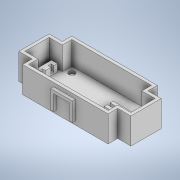
# Autodesk Inventor part: Final Design
Saved by Autodesk Inventor 2021 (Build 250183000, 183)
## iProperties
Created: 2020-11-11
Part Number: Final Design
Material: Generic
Document SubType Name: Modeling
Designer: coupe
Density: 1 g/cm^3
Appearance: Default
Mass: 94.4027 g
Surface Area: 493.885 cm^2
Volume: 94.4027 cm^3
Author: coupe
Autodesk Inventor part; units mm, degrees
ref_plane "YZ Plane" through (0, 0, 0) normal (1, 0, 0) x (0, 1, 0)
ref_plane "XZ Plane" through (0, 0, 0) normal (0, 1, 0) x (-1, 0, 0)
sketch "Sketch1" plane through (0, 0, 0) normal (0, 0, 1) x (1, 0, 0)
  line L0 (0, 0) -> (150.4, 0)
  line L1 (150.4, 0) -> (150.4, 35)
  line L2 (150.4, 35) -> (0, 35)
  line L3 (0, 35) -> (0, 0)
  line L4 (0, 35) -> (17.78, 35)
  line L5 (17.78, 0) -> (0, 0)
  line L6 (0, 0) -> (0, 35)
  line L7 (150.4, 0) -> (134.62, 0)
  line L8 (134.62, 35) -> (150.4, 35)
  line L9 (150.4, 35) -> (150.4, 0)
  dimension "d0" = 150.4
  dimension "d1" = 35
  constraints: 20 end point, 4 parallel, 3 horizontal, 2 point on line, 1 perpendicular
  measures "d0" distance between parallel lines of L3 L1
  measures "d1" distance between parallel lines of L0 L2
extrude "Extrusion1" add sketch "Sketch1" against normal blind 33.1
sketch "Sketch2" plane through (0, 0, 0) normal (0, 0, 1) x (1, 0, 0)
  line L0 (0, 35) -> (150.4, 35) projected
  line L1 (150.4, 0) -> (0, 0) projected
  line L2 (0, 35) -> (17.78, 35)
  line L3 (17.78, 35) -> (17.78, 0)
  line L4 (17.78, 0) -> (0, 0)
  line L5 (0, 0) -> (0, 35)
  line L6 (150.4, 0) -> (132.62, 0)
  line L7 (132.62, 0) -> (132.62, 35)
  line L8 (132.62, 35) -> (150.4, 35)
  line L9 (150.4, 35) -> (150.4, 0)
  point P0 (132.62, 0)
  dimension "d6" = 17.78
  dimension "d7" = 17.78
  constraints: 16 end point, 4 parallel, 2 horizontal, 2 perpendicular, 2 point on line
  measures "d6" distance between parallel lines of L5 L3
  measures "d7" distance between parallel lines of L9 L7
extrude "Extrusion2" cut sketch "Sketch2" against normal blind 12.8 contours L0 L3 L1 L5 | L0 L9 L1 L7
shell "Shell1" thickness 4 removed faces 2 at (94.34, 35, -26.3333) at (100.2667, 11.6667, -33.1)
sketch "Sketch3" plane through (0, 0, 0) normal (0, 0, 1) x (1, 0, 0)
  line L0 (59.55, 30) -> (88.85, 30)
  line L1 (88.85, 30) -> (88.85, 5)
  line L2 (88.85, 5) -> (59.55, 5)
  line L3 (59.55, 5) -> (59.55, 30)
  line L4 (132.62, 35) -> (17.78, 35) projected
  line L5 (132.62, 0) -> (132.62, 35) projected
  point P0 (0, 0)
  dimension "d11" = 5
  dimension "d12" = 43.77
  dimension "d13" = 25
  dimension "d14" = 29.3
  constraints: 8 end point, 2 parallel, 1 horizontal, 1 perpendicular
  measures "d11" distance between parallel lines of L4 L0
  measures "d12" distance between parallel lines of L5 L1
  measures "d13" distance between parallel lines of L0 L2
  measures "d14" distance between parallel lines of L1 L3
extrude "Extrusion3" add sketch "Sketch3" along normal blind 4
shell "Shell2" thickness 4 removed faces 1 at (69.3167, 21.6667, 4)
sketch "Sketch5" plane through (0, 0, 4) normal (0, 0, 1) x (1, 0, 0)
  line L0 (63.55, 9) -> (84.85, 9) projected
  line L1 (88.85, 5) -> (59.55, 5) projected
  line L2 (63.55, 9) -> (84.85, 9)
  line L3 (84.85, 9) -> (84.85, 5)
  line L4 (84.85, 5) -> (63.55, 5)
  line L5 (63.55, 5) -> (63.55, 9)
  point P0 (0, 0)
  point P1 (63.55, 5)
  dimension "d18" = 21.3
  constraints: 8 end point, 2 parallel, 1 horizontal, 1 perpendicular, 1 point on line
  measures "d18" distance between parallel lines of L5 L3
extrude "Extrusion4" cut sketch "Sketch5" against normal blind 4
ref_plane "Work Plane2" through (0, 0, -33.1) normal (0, 0, 1) x (1, 0, 0)
mirror "Mirror1" about plane through (0, 0, -33.1) normal (0, 0, 1)
sketch "Sketch10" plane through (21.78, 4, -4) normal (0, 1, 0) x (1, 0, 0)
  line L0 (-10.705, 22.1) -> (117.545, 22.1)
  line L1 (117.545, 22.1) -> (117.545, 36.1)
  line L2 (117.545, 36.1) -> (-10.705, 36.1)
  line L3 (-10.705, 36.1) -> (-10.705, 22.1)
  line L4 (124.62, 45.4) -> (106.84, 45.4) projected
  line L5 (124.62, 12.8) -> (106.84, 12.8) projected
  line L6 (-17.78, 12.8) -> (-17.78, 45.4) projected
  line L7 (124.62, 45.4) -> (124.62, 12.8) projected
  line L8 (117.545, 23.1) -> (78.545, 23.1)
  line L9 (78.545, 23.1) -> (78.545, 35.1)
  line L10 (78.545, 35.1) -> (117.545, 35.1)
  line L11 (117.545, 35.1) -> (117.545, 23.1)
  line L12 (-10.705, 22.1) -> (-4.955, 22.1)
  line L13 (-10.705, 31.1) -> (-10.705, 22.1)
  line L14 (-10.705, 16.8) -> (-2.705, 16.8)
  line L15 (-10.705, 27.6) -> (-10.705, 16.8)
  line L16 (-10.705, 41.4) -> (-2.705, 41.4)
  line L17 (-2.705, 41.4) -> (-2.705, 16.8)
  line L18 (-10.705, 30.6) -> (-10.705, 41.4)
  point P0 (-21.78, -4)
  point P1 (117.545, 29.1)
  point P2 (-2.705, 36.1)
  point P3 (-2.705, 22.1)
  point P4 (-10.705, 36.1)
  dimension "d27" = 9.3
  dimension "d28" = 9.3
  dimension "d29" = 7.075
  dimension "d30" = 7.075
  dimension "d31" = 12
  dimension "d32" = 6
  dimension "d33" = 39
  dimension "d36" = 5.3
  dimension "d39" = 7.075
  dimension "d41" = 5.3
  dimension "d42" = 8
  constraints: 30 end point, 5 horizontal, 5 parallel, 3 perpendicular, 2 coincident, 2 point on line, 1 midpoint
  measures "d27" distance between parallel lines of L4 L2
  measures "d28" distance between parallel lines of L5 L0
  measures "d29" distance between parallel lines of L6 L3
  measures "d30" distance between parallel lines of L7 L1
  measures "d31" distance between parallel lines of L10 L8
  measures "d32" distance from line of point (117.545, 29.1) L10
  measures "d33" distance between parallel lines of L11 L9
  measures "d36" distance between parallel lines of L0 L14
  measures "d39" distance between parallel lines of L6 L15
  measures "d41" distance between parallel lines of L2 L16
  measures "d42" distance between parallel lines of L18 L17
extrude "Extrusion5" add sketch "Sketch10" along normal blind 10 contours L3 L2 L17 L0 | L0 L17 L14 L15 | L2 L18 L16 L17 | L8 L9 L10 L1
shell "Shell5" thickness 4 removed faces 2 at (126.325, 14, -35.1) at (100.325, 7.3333, -35.1)
sketch "Sketch12" plane through (21.78, 14, -4) normal (0, 1, 0) x (1, 0, 0)
  line L0 (-2.705, 41.4) -> (-2.705, 16.8)
  line L1 (-2.705, 36.598) -> (-2.705, 32.6553)
  line L2 (-10.705, 41.4) -> (-10.705, 16.8)
  line L3 (-2.705, 41.4) -> (-10.705, 41.4)
  line L4 (-2.705, 32.6553) -> (-6.705, 32.9)
  line L5 (-6.705, 32.9) -> (-6.705, 36.9)
  line L6 (-6.705, 36.9) -> (-2.705, 36.6553)
  line L7 (-2.705, 36.598) -> (-2.705, 36.6553)
  line L8 (-10.705, 41.4) -> (-10.705, 16.8)
  line L9 (-2.705, 16.8) -> (-2.705, 27.6)
  line L10 (-2.705, 22.2) -> (-2.705, 21.5447)
  line L11 (-2.705, 21.5447) -> (-6.705, 21.3)
  line L12 (-6.705, 21.3) -> (-6.705, 25.3)
  line L13 (-6.705, 25.3) -> (-2.705, 25.5447)
  line L14 (-2.705, 25.5447) -> (-2.705, 21.5447)
  line L15 (-10.705, 16.8) -> (-2.705, 16.8) projected
  point P0 (-21.78, -4)
  point P1 (-1.955, 30.6)
  point P2 (-9.955, 30.6)
  dimension "d51" = 93.5
  dimension "d60" = 86.5
  dimension "d63" = 93.5
  dimension "d64" = 4
  dimension "d65" = 4
  dimension "d66" = 4
  dimension "d67" = 4
  dimension "d68" = 24.6
  dimension "d69" = 4.5
  dimension "d70" = 4.5
  constraints: 26 end point, 2 point on line, 1 midpoint, 1 parallel, 8 other
  measures "d60" angle of L9 L11
  measures "d63" angle of L9 L13
  measures "d64" length of L12
  measures "d65" distance between parallel lines of L8 L5
  measures "d66" distance of L11.end L12.end
  measures "d67" distance of L5.end L4.end
  measures "d68" distance between parallel lines of L3 L15
  measures "d69" distance from line of L15 L11.end
  measures "d70" distance from line of L3 L5.end
extrude "Extrusion6" cut sketch "Sketch12" against normal blind 7.5 contours L0 L4 L5 L6 | L11 L12 L13 L0
sketch "Sketch19" plane through (21.78, 4, -62.2) normal (0, 1, 0) x (1, 0, 0)
  circle A0 centre (8, -8) radius 4
  line L0 (106.84, 0) -> (0, 0) projected
  line L1 (0, 0) -> (0, -12.8) projected
  circle A1 centre (8, -50.2) radius 4
  circle A2 centre (98.84, -8) radius 4
  circle A3 centre (98.84, -50.2) radius 4
  line L2 (106.84, -58.2) -> (0, -58.2) projected
  line L3 (0, -58.2) -> (0, -45.4) projected
  line L4 (106.84, -12.8) -> (106.84, 0) projected
  line L5 (106.84, -45.4) -> (106.84, -58.2) projected
  point P0 (-21.78, -62.2)
  dimension "d126" = 8
  dimension "d127" = 4
  dimension "d128" = 4
  dimension "d129" = 8
  dimension "d130" = 4
  dimension "d131" = 4
  dimension "d132" = 8
  dimension "d133" = 4
  dimension "d134" = 4
  dimension "d135" = 8
  dimension "d136" = 4
  dimension "d137" = 4
  constraints: 4 centre point
  measures "d126" diameter of A0
  measures "d127" distance edge to line of A0 L0
  measures "d128" distance edge to line of A0 L1
  measures "d129" diameter of A1
  measures "d130" distance edge to line of A1 L2
  measures "d131" distance edge to line of A1 L3
  measures "d132" diameter of A2
  measures "d133" distance edge to line of A2 L0
  measures "d134" distance edge to line of A2 L4
  measures "d135" diameter of A3
  measures "d136" distance edge to line of A3 L5
  measures "d137" distance edge to line of A3 L2
extrude "Extrusion12" cut sketch "Sketch19" against normal blind 10
body "Solid1"
